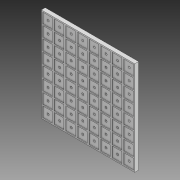
# Autodesk Inventor part: Solenoid Plate
Saved by Autodesk Inventor 2020 (Build 240168000, 168)
## iProperties
Created: 2020-08-11
Part Number: Solenoid Plate
Material: Generic
Document SubType Name: Modeling
Designer: DDeGo
Density: 1 g/cm^3
Appearance: Default
Author: DDeGo
Autodesk Inventor part; units mm, degrees
ref_plane "YZ Plane" through (0, 0, 0) normal (1, 0, 0) x (0, 1, 0)
ref_plane "XZ Plane" through (0, 0, 0) normal (0, 1, 0) x (-1, 0, 0)
ref_plane "XY Plane" through (0, 0, 0) normal (0, 0, 1) x (1, 0, 0)
sketch "Sketch1" plane through (0, 0, 0) normal (0, 0, 1) x (1, 0, 0)
  line L0 (0, 0) -> (145, 0)
  line L1 (145, 0) -> (145, 146)
  line L2 (145, 146) -> (0, 146)
  line L3 (0, 146) -> (0, 0)
  line L4 (2, 2) -> (17, 2) construction
  line L5 (17, 2) -> (17, 18) construction
  line L6 (17, 18) -> (2, 18) construction
  line L7 (2, 18) -> (2, 2) construction
  line L8 (2, 2) -> (17, 18) construction
  line L9 (17, 2) -> (2, 18) construction
  circle A0 centre (9.5, 10) radius 1.6
  line L10 (20, 2) -> (35, 2) construction
  line L11 (35, 2) -> (35, 18) construction
  line L12 (35, 18) -> (20, 18) construction
  line L13 (20, 18) -> (20, 2) construction
  line L14 (20, 2) -> (35, 18) construction
  line L15 (35, 2) -> (20, 18) construction
  circle A1 centre (27.5, 10) radius 1.6
  line L16 (38, 2) -> (53, 2) construction
  line L17 (53, 2) -> (53, 18) construction
  line L18 (53, 18) -> (38, 18) construction
  line L19 (38, 18) -> (38, 2) construction
  line L20 (38, 2) -> (53, 18) construction
  line L21 (53, 2) -> (38, 18) construction
  circle A2 centre (45.5, 10) radius 1.6
  line L22 (56, 2) -> (71, 2) construction
  line L23 (71, 2) -> (71, 18) construction
  line L24 (71, 18) -> (56, 18) construction
  line L25 (56, 18) -> (56, 2) construction
  line L26 (56, 2) -> (71, 18) construction
  line L27 (71, 2) -> (56, 18) construction
  circle A3 centre (63.5, 10) radius 1.6
  line L28 (74, 2) -> (89, 2) construction
  line L29 (89, 2) -> (89, 18) construction
  line L30 (89, 18) -> (74, 18) construction
  line L31 (74, 18) -> (74, 2) construction
  line L32 (74, 2) -> (89, 18) construction
  line L33 (89, 2) -> (74, 18) construction
  circle A4 centre (81.5, 10) radius 1.6
  line L34 (92, 2) -> (107, 2) construction
  line L35 (107, 2) -> (107, 18) construction
  line L36 (107, 18) -> (92, 18) construction
  line L37 (92, 18) -> (92, 2) construction
  line L38 (92, 2) -> (107, 18) construction
  line L39 (107, 2) -> (92, 18) construction
  circle A5 centre (99.5, 10) radius 1.6
  line L40 (110, 2) -> (125, 2) construction
  line L41 (125, 2) -> (125, 18) construction
  line L42 (125, 18) -> (110, 18) construction
  line L43 (110, 18) -> (110, 2) construction
  line L44 (110, 2) -> (125, 18) construction
  line L45 (125, 2) -> (110, 18) construction
  circle A6 centre (117.5, 10) radius 1.6
  line L46 (128, 2) -> (143, 2) construction
  line L47 (143, 2) -> (143, 18) construction
  line L48 (143, 18) -> (128, 18) construction
  line L49 (128, 18) -> (128, 2) construction
  line L50 (128, 2) -> (143, 18) construction
  line L51 (143, 2) -> (128, 18) construction
  circle A7 centre (135.5, 10) radius 1.6
  line L52 (2, 20) -> (17, 20) construction
  line L53 (17, 20) -> (17, 36) construction
  line L54 (17, 36) -> (2, 36) construction
  line L55 (2, 36) -> (2, 20) construction
  line L56 (2, 20) -> (17, 36) construction
  line L57 (17, 20) -> (2, 36) construction
  circle A8 centre (9.5, 28) radius 1.6
  line L58 (20, 20) -> (35, 20) construction
  line L59 (35, 20) -> (35, 36) construction
  line L60 (35, 36) -> (20, 36) construction
  line L61 (20, 36) -> (20, 20) construction
  line L62 (20, 20) -> (35, 36) construction
  line L63 (35, 20) -> (20, 36) construction
  circle A9 centre (27.5, 28) radius 1.6
  line L64 (38, 20) -> (53, 20) construction
  line L65 (53, 20) -> (53, 36) construction
  line L66 (53, 36) -> (38, 36) construction
  line L67 (38, 36) -> (38, 20) construction
  line L68 (38, 20) -> (53, 36) construction
  line L69 (53, 20) -> (38, 36) construction
  circle A10 centre (45.5, 28) radius 1.6
  line L70 (56, 20) -> (71, 20) construction
  line L71 (71, 20) -> (71, 36) construction
  line L72 (71, 36) -> (56, 36) construction
  line L73 (56, 36) -> (56, 20) construction
  line L74 (56, 20) -> (71, 36) construction
  line L75 (71, 20) -> (56, 36) construction
  circle A11 centre (63.5, 28) radius 1.6
  line L76 (74, 20) -> (89, 20) construction
  line L77 (89, 20) -> (89, 36) construction
  line L78 (89, 36) -> (74, 36) construction
  line L79 (74, 36) -> (74, 20) construction
  line L80 (74, 20) -> (89, 36) construction
  line L81 (89, 20) -> (74, 36) construction
  circle A12 centre (81.5, 28) radius 1.6
  line L82 (92, 20) -> (107, 20) construction
  line L83 (107, 20) -> (107, 36) construction
  line L84 (107, 36) -> (92, 36) construction
  line L85 (92, 36) -> (92, 20) construction
  line L86 (92, 20) -> (107, 36) construction
  line L87 (107, 20) -> (92, 36) construction
  circle A13 centre (99.5, 28) radius 1.6
  line L88 (110, 20) -> (125, 20) construction
  line L89 (125, 20) -> (125, 36) construction
  line L90 (125, 36) -> (110, 36) construction
  line L91 (110, 36) -> (110, 20) construction
  line L92 (110, 20) -> (125, 36) construction
  line L93 (125, 20) -> (110, 36) construction
  circle A14 centre (117.5, 28) radius 1.6
  line L94 (128, 20) -> (143, 20) construction
  line L95 (143, 20) -> (143, 36) construction
  line L96 (143, 36) -> (128, 36) construction
  line L97 (128, 36) -> (128, 20) construction
  line L98 (128, 20) -> (143, 36) construction
  line L99 (143, 20) -> (128, 36) construction
  circle A15 centre (135.5, 28) radius 1.6
  line L100 (2, 38) -> (17, 38) construction
  line L101 (17, 38) -> (17, 54) construction
  line L102 (17, 54) -> (2, 54) construction
  line L103 (2, 54) -> (2, 38) construction
  line L104 (2, 38) -> (17, 54) construction
  line L105 (17, 38) -> (2, 54) construction
  circle A16 centre (9.5, 46) radius 1.6
  line L106 (20, 38) -> (35, 38) construction
  line L107 (35, 38) -> (35, 54) construction
  line L108 (35, 54) -> (20, 54) construction
  line L109 (20, 54) -> (20, 38) construction
  line L110 (20, 38) -> (35, 54) construction
  line L111 (35, 38) -> (20, 54) construction
  circle A17 centre (27.5, 46) radius 1.6
  line L112 (38, 38) -> (53, 38) construction
  line L113 (53, 38) -> (53, 54) construction
  line L114 (53, 54) -> (38, 54) construction
  line L115 (38, 54) -> (38, 38) construction
  line L116 (38, 38) -> (53, 54) construction
  line L117 (53, 38) -> (38, 54) construction
  circle A18 centre (45.5, 46) radius 1.6
  line L118 (56, 38) -> (71, 38) construction
  line L119 (71, 38) -> (71, 54) construction
  line L120 (71, 54) -> (56, 54) construction
  line L121 (56, 54) -> (56, 38) construction
  line L122 (56, 38) -> (71, 54) construction
  line L123 (71, 38) -> (56, 54) construction
  circle A19 centre (63.5, 46) radius 1.6
  line L124 (74, 38) -> (89, 38) construction
  line L125 (89, 38) -> (89, 54) construction
  line L126 (89, 54) -> (74, 54) construction
  line L127 (74, 54) -> (74, 38) construction
  line L128 (74, 38) -> (89, 54) construction
  line L129 (89, 38) -> (74, 54) construction
  circle A20 centre (81.5, 46) radius 1.6
  line L130 (92, 38) -> (107, 38) construction
  line L131 (107, 38) -> (107, 54) construction
  line L132 (107, 54) -> (92, 54) construction
  line L133 (92, 54) -> (92, 38) construction
  line L134 (92, 38) -> (107, 54) construction
  line L135 (107, 38) -> (92, 54) construction
  circle A21 centre (99.5, 46) radius 1.6
  line L136 (110, 38) -> (125, 38) construction
  line L137 (125, 38) -> (125, 54) construction
  line L138 (125, 54) -> (110, 54) construction
  line L139 (110, 54) -> (110, 38) construction
  line L140 (110, 38) -> (125, 54) construction
  line L141 (125, 38) -> (110, 54) construction
  circle A22 centre (117.5, 46) radius 1.6
  line L142 (128, 38) -> (143, 38) construction
  line L143 (143, 38) -> (143, 54) construction
  line L144 (143, 54) -> (128, 54) construction
  line L145 (128, 54) -> (128, 38) construction
  line L146 (128, 38) -> (143, 54) construction
  line L147 (143, 38) -> (128, 54) construction
  circle A23 centre (135.5, 46) radius 1.6
  line L148 (2, 56) -> (17, 56) construction
  line L149 (17, 56) -> (17, 72) construction
  line L150 (17, 72) -> (2, 72) construction
  line L151 (2, 72) -> (2, 56) construction
  line L152 (2, 56) -> (17, 72) construction
  line L153 (17, 56) -> (2, 72) construction
  circle A24 centre (9.5, 64) radius 1.6
  line L154 (20, 56) -> (35, 56) construction
  line L155 (35, 56) -> (35, 72) construction
  line L156 (35, 72) -> (20, 72) construction
  line L157 (20, 72) -> (20, 56) construction
  line L158 (20, 56) -> (35, 72) construction
  line L159 (35, 56) -> (20, 72) construction
  circle A25 centre (27.5, 64) radius 1.6
  line L160 (38, 56) -> (53, 56) construction
  line L161 (53, 56) -> (53, 72) construction
  line L162 (53, 72) -> (38, 72) construction
  line L163 (38, 72) -> (38, 56) construction
  line L164 (38, 56) -> (53, 72) construction
  line L165 (53, 56) -> (38, 72) construction
  circle A26 centre (45.5, 64) radius 1.6
  line L166 (56, 56) -> (71, 56) construction
  line L167 (71, 56) -> (71, 72) construction
  line L168 (71, 72) -> (56, 72) construction
  line L169 (56, 72) -> (56, 56) construction
  line L170 (56, 56) -> (71, 72) construction
  line L171 (71, 56) -> (56, 72) construction
  circle A27 centre (63.5, 64) radius 1.6
  line L172 (74, 56) -> (89, 56) construction
  line L173 (89, 56) -> (89, 72) construction
  line L174 (89, 72) -> (74, 72) construction
  line L175 (74, 72) -> (74, 56) construction
  line L176 (74, 56) -> (89, 72) construction
  line L177 (89, 56) -> (74, 72) construction
  circle A28 centre (81.5, 64) radius 1.6
  line L178 (92, 56) -> (107, 56) construction
  line L179 (107, 56) -> (107, 72) construction
  line L180 (107, 72) -> (92, 72) construction
  line L181 (92, 72) -> (92, 56) construction
  line L182 (92, 56) -> (107, 72) construction
  line L183 (107, 56) -> (92, 72) construction
  circle A29 centre (99.5, 64) radius 1.6
  line L184 (110, 56) -> (125, 56) construction
  line L185 (125, 56) -> (125, 72) construction
  line L186 (125, 72) -> (110, 72) construction
  line L187 (110, 72) -> (110, 56) construction
  line L188 (110, 56) -> (125, 72) construction
  line L189 (125, 56) -> (110, 72) construction
  circle A30 centre (117.5, 64) radius 1.6
  line L190 (128, 56) -> (143, 56) construction
  line L191 (143, 56) -> (143, 72) construction
  line L192 (143, 72) -> (128, 72) construction
  line L193 (128, 72) -> (128, 56) construction
  line L194 (128, 56) -> (143, 72) construction
  line L195 (143, 56) -> (128, 72) construction
  circle A31 centre (135.5, 64) radius 1.6
  line L196 (2, 74) -> (17, 74) construction
  line L197 (17, 74) -> (17, 90) construction
  line L198 (17, 90) -> (2, 90) construction
  line L199 (2, 90) -> (2, 74) construction
  line L200 (2, 74) -> (17, 90) construction
  line L201 (17, 74) -> (2, 90) construction
  circle A32 centre (9.5, 82) radius 1.6
  line L202 (20, 74) -> (35, 74) construction
  line L203 (35, 74) -> (35, 90) construction
  line L204 (35, 90) -> (20, 90) construction
  line L205 (20, 90) -> (20, 74) construction
  line L206 (20, 74) -> (35, 90) construction
  line L207 (35, 74) -> (20, 90) construction
  circle A33 centre (27.5, 82) radius 1.6
  line L208 (38, 74) -> (53, 74) construction
  line L209 (53, 74) -> (53, 90) construction
  line L210 (53, 90) -> (38, 90) construction
  line L211 (38, 90) -> (38, 74) construction
  line L212 (38, 74) -> (53, 90) construction
  line L213 (53, 74) -> (38, 90) construction
  circle A34 centre (45.5, 82) radius 1.6
  line L214 (56, 74) -> (71, 74) construction
  line L215 (71, 74) -> (71, 90) construction
  line L216 (71, 90) -> (56, 90) construction
  line L217 (56, 90) -> (56, 74) construction
  line L218 (56, 74) -> (71, 90) construction
  line L219 (71, 74) -> (56, 90) construction
  circle A35 centre (63.5, 82) radius 1.6
  line L220 (74, 74) -> (89, 74) construction
  line L221 (89, 74) -> (89, 90) construction
  line L222 (89, 90) -> (74, 90) construction
  line L223 (74, 90) -> (74, 74) construction
  line L224 (74, 74) -> (89, 90) construction
  line L225 (89, 74) -> (74, 90) construction
  circle A36 centre (81.5, 82) radius 1.6
  line L226 (92, 74) -> (107, 74) construction
  line L227 (107, 74) -> (107, 90) construction
  line L228 (107, 90) -> (92, 90) construction
  line L229 (92, 90) -> (92, 74) construction
  line L230 (92, 74) -> (107, 90) construction
  line L231 (107, 74) -> (92, 90) construction
  circle A37 centre (99.5, 82) radius 1.6
  line L232 (110, 74) -> (125, 74) construction
  line L233 (125, 74) -> (125, 90) construction
  line L234 (125, 90) -> (110, 90) construction
  line L235 (110, 90) -> (110, 74) construction
  line L236 (110, 74) -> (125, 90) construction
  line L237 (125, 74) -> (110, 90) construction
  circle A38 centre (117.5, 82) radius 1.6
  line L238 (128, 74) -> (143, 74) construction
  line L239 (143, 74) -> (143, 90) construction
  line L240 (143, 90) -> (128, 90) construction
  line L241 (128, 90) -> (128, 74) construction
  line L242 (128, 74) -> (143, 90) construction
  line L243 (143, 74) -> (128, 90) construction
  circle A39 centre (135.5, 82) radius 1.6
  line L244 (2, 92) -> (17, 92) construction
  line L245 (17, 92) -> (17, 108) construction
  line L246 (17, 108) -> (2, 108) construction
  line L247 (2, 108) -> (2, 92) construction
  line L248 (2, 92) -> (17, 108) construction
  line L249 (17, 92) -> (2, 108) construction
  circle A40 centre (9.5, 100) radius 1.6
  line L250 (20, 92) -> (35, 92) construction
  line L251 (35, 92) -> (35, 108) construction
  line L252 (35, 108) -> (20, 108) construction
  line L253 (20, 108) -> (20, 92) construction
  line L254 (20, 92) -> (35, 108) construction
  line L255 (35, 92) -> (20, 108) construction
  circle A41 centre (27.5, 100) radius 1.6
  line L256 (38, 92) -> (53, 92) construction
  line L257 (53, 92) -> (53, 108) construction
  line L258 (53, 108) -> (38, 108) construction
  line L259 (38, 108) -> (38, 92) construction
  line L260 (38, 92) -> (53, 108) construction
  line L261 (53, 92) -> (38, 108) construction
  circle A42 centre (45.5, 100) radius 1.6
  line L262 (56, 92) -> (71, 92) construction
  line L263 (71, 92) -> (71, 108) construction
  line L264 (71, 108) -> (56, 108) construction
  line L265 (56, 108) -> (56, 92) construction
  line L266 (56, 92) -> (71, 108) construction
  line L267 (71, 92) -> (56, 108) construction
  circle A43 centre (63.5, 100) radius 1.6
  line L268 (74, 92) -> (89, 92) construction
  line L269 (89, 92) -> (89, 108) construction
  line L270 (89, 108) -> (74, 108) construction
  line L271 (74, 108) -> (74, 92) construction
  line L272 (74, 92) -> (89, 108) construction
  line L273 (89, 92) -> (74, 108) construction
  circle A44 centre (81.5, 100) radius 1.6
  line L274 (92, 92) -> (107, 92) construction
  line L275 (107, 92) -> (107, 108) construction
  line L276 (107, 108) -> (92, 108) construction
  line L277 (92, 108) -> (92, 92) construction
  line L278 (92, 92) -> (107, 108) construction
  line L279 (107, 92) -> (92, 108) construction
  circle A45 centre (99.5, 100) radius 1.6
  line L280 (110, 92) -> (125, 92) construction
  line L281 (125, 92) -> (125, 108) construction
  line L282 (125, 108) -> (110, 108) construction
  line L283 (110, 108) -> (110, 92) construction
  line L284 (110, 92) -> (125, 108) construction
  line L285 (125, 92) -> (110, 108) construction
  circle A46 centre (117.5, 100) radius 1.6
  line L286 (128, 92) -> (143, 92) construction
  line L287 (143, 92) -> (143, 108) construction
  line L288 (143, 108) -> (128, 108) construction
  line L289 (128, 108) -> (128, 92) construction
  line L290 (128, 92) -> (143, 108) construction
  line L291 (143, 92) -> (128, 108) construction
  circle A47 centre (135.5, 100) radius 1.6
  line L292 (2, 110) -> (17, 110) construction
  line L293 (17, 110) -> (17, 126) construction
  line L294 (17, 126) -> (2, 126) construction
  line L295 (2, 126) -> (2, 110) construction
  line L296 (2, 110) -> (17, 126) construction
  line L297 (17, 110) -> (2, 126) construction
  circle A48 centre (9.5, 118) radius 1.6
  line L298 (20, 110) -> (35, 110) construction
  line L299 (35, 110) -> (35, 126) construction
  line L300 (35, 126) -> (20, 126) construction
  line L301 (20, 126) -> (20, 110) construction
  line L302 (20, 110) -> (35, 126) construction
  line L303 (35, 110) -> (20, 126) construction
  circle A49 centre (27.5, 118) radius 1.6
  line L304 (38, 110) -> (53, 110) construction
  line L305 (53, 110) -> (53, 126) construction
  line L306 (53, 126) -> (38, 126) construction
  line L307 (38, 126) -> (38, 110) construction
  line L308 (38, 110) -> (53, 126) construction
  line L309 (53, 110) -> (38, 126) construction
  circle A50 centre (45.5, 118) radius 1.6
  line L310 (56, 110) -> (71, 110) construction
  line L311 (71, 110) -> (71, 126) construction
  line L312 (71, 126) -> (56, 126) construction
  line L313 (56, 126) -> (56, 110) construction
  line L314 (56, 110) -> (71, 126) construction
  line L315 (71, 110) -> (56, 126) construction
  circle A51 centre (63.5, 118) radius 1.6
  line L316 (74, 110) -> (89, 110) construction
  line L317 (89, 110) -> (89, 126) construction
  line L318 (89, 126) -> (74, 126) construction
  line L319 (74, 126) -> (74, 110) construction
  line L320 (74, 110) -> (89, 126) construction
  line L321 (89, 110) -> (74, 126) construction
  circle A52 centre (81.5, 118) radius 1.6
  line L322 (92, 110) -> (107, 110) construction
  line L323 (107, 110) -> (107, 126) construction
  line L324 (107, 126) -> (92, 126) construction
  line L325 (92, 126) -> (92, 110) construction
  line L326 (92, 110) -> (107, 126) construction
  line L327 (107, 110) -> (92, 126) construction
  circle A53 centre (99.5, 118) radius 1.6
  line L328 (110, 110) -> (125, 110) construction
  line L329 (125, 110) -> (125, 126) construction
  line L330 (125, 126) -> (110, 126) construction
  line L331 (110, 126) -> (110, 110) construction
  line L332 (110, 110) -> (125, 126) construction
  line L333 (125, 110) -> (110, 126) construction
  circle A54 centre (117.5, 118) radius 1.6
  line L334 (128, 110) -> (143, 110) construction
  line L335 (143, 110) -> (143, 126) construction
  line L336 (143, 126) -> (128, 126) construction
  line L337 (128, 126) -> (128, 110) construction
  line L338 (128, 110) -> (143, 126) construction
  line L339 (143, 110) -> (128, 126) construction
  circle A55 centre (135.5, 118) radius 1.6
  line L340 (2, 128) -> (17, 128) construction
  line L341 (17, 128) -> (17, 144) construction
  line L342 (17, 144) -> (2, 144) construction
  line L343 (2, 144) -> (2, 128) construction
  line L344 (2, 128) -> (17, 144) construction
  line L345 (17, 128) -> (2, 144) construction
  circle A56 centre (9.5, 136) radius 1.6
  line L346 (20, 128) -> (35, 128) construction
  line L347 (35, 128) -> (35, 144) construction
  line L348 (35, 144) -> (20, 144) construction
  line L349 (20, 144) -> (20, 128) construction
  line L350 (20, 128) -> (35, 144) construction
  line L351 (35, 128) -> (20, 144) construction
  circle A57 centre (27.5, 136) radius 1.6
  line L352 (38, 128) -> (53, 128) construction
  line L353 (53, 128) -> (53, 144) construction
  line L354 (53, 144) -> (38, 144) construction
  line L355 (38, 144) -> (38, 128) construction
  line L356 (38, 128) -> (53, 144) construction
  line L357 (53, 128) -> (38, 144) construction
  circle A58 centre (45.5, 136) radius 1.6
  line L358 (56, 128) -> (71, 128) construction
  line L359 (71, 128) -> (71, 144) construction
  line L360 (71, 144) -> (56, 144) construction
  line L361 (56, 144) -> (56, 128) construction
  line L362 (56, 128) -> (71, 144) construction
  line L363 (71, 128) -> (56, 144) construction
  circle A59 centre (63.5, 136) radius 1.6
  line L364 (74, 128) -> (89, 128) construction
  line L365 (89, 128) -> (89, 144) construction
  line L366 (89, 144) -> (74, 144) construction
  line L367 (74, 144) -> (74, 128) construction
  line L368 (74, 128) -> (89, 144) construction
  line L369 (89, 128) -> (74, 144) construction
  circle A60 centre (81.5, 136) radius 1.6
  line L370 (92, 128) -> (107, 128) construction
  line L371 (107, 128) -> (107, 144) construction
  line L372 (107, 144) -> (92, 144) construction
  line L373 (92, 144) -> (92, 128) construction
  line L374 (92, 128) -> (107, 144) construction
  line L375 (107, 128) -> (92, 144) construction
  circle A61 centre (99.5, 136) radius 1.6
  line L376 (110, 128) -> (125, 128) construction
  line L377 (125, 128) -> (125, 144) construction
  line L378 (125, 144) -> (110, 144) construction
  line L379 (110, 144) -> (110, 128) construction
  line L380 (110, 128) -> (125, 144) construction
  line L381 (125, 128) -> (110, 144) construction
  circle A62 centre (117.5, 136) radius 1.6
  line L382 (128, 128) -> (143, 128) construction
  line L383 (143, 128) -> (143, 144) construction
  line L384 (143, 144) -> (128, 144) construction
  line L385 (128, 144) -> (128, 128) construction
  line L386 (128, 128) -> (143, 144) construction
  line L387 (143, 128) -> (128, 144) construction
  circle A63 centre (135.5, 136) radius 1.6
  point P0 (9.5, 10)
  point P1 (27.5, 10)
  point P2 (45.5, 10)
  point P3 (63.5, 10)
  point P4 (81.5, 10)
  point P5 (99.5, 10)
  point P6 (117.5, 10)
  point P7 (135.5, 10)
  point P8 (9.5, 28)
  point P9 (63.5, 28)
  point P10 (9.5, 46)
  point P11 (63.5, 46)
  point P12 (9.5, 64)
  point P13 (63.5, 64)
  point P14 (9.5, 82)
  point P15 (63.5, 82)
  point P16 (9.5, 100)
  point P17 (63.5, 100)
  point P18 (9.5, 118)
  point P19 (63.5, 118)
  point P20 (9.5, 136)
  point P21 (63.5, 136)
  dimension "d0" = 2
  dimension "d1" = 2
  dimension "d2" = 16
  dimension "d3" = 15
  dimension "d4" = 3.2
  dimension "d7" = 18
  dimension "d10" = 18
  dimension "d13" = 2
  dimension "d14" = 2
  dimension "d27" = 145
  dimension "d28" = 146
  constraints: 776 end point, 128 midpoint, 64 centre point, 64 coincident, 4 parallel, 3 horizontal, 2 perpendicular, 1 vertical, 819 other
  measures "d0" distance between parallel lines of L0 L4
  measures "d1" distance between parallel lines of L3 L7
  measures "d2" distance of L6.end L4.start
  measures "d3" distance of L4.start L4.end
  measures "d4" diameter of A0
  measures "d7" distance of L4.start L10.start
  measures "d10" distance of L4.start L52.start
  measures "d13" distance between parallel lines of L1 L47
  measures "d14" distance between parallel lines of L2 L342
  measures "d27" distance of L1.end L2.end
  measures "d28" distance of L0.end L1.end
extrude "Extrusion1" add sketch "Sketch1" along normal blind 6
sketch "Sketch2" plane through (0, 0, 6) normal (0, 0, 1) x (1, 0, 0)
  line L0 (2, 2) -> (17, 2)
  line L1 (17, 2) -> (17, 18)
  line L2 (17, 18) -> (2, 18)
  line L3 (2, 18) -> (2, 2)
  line L4 (2, 2) -> (17, 18) construction
  line L5 (17, 2) -> (2, 18) construction
  line L6 (20, 2) -> (35, 2)
  line L7 (35, 2) -> (35, 18)
  line L8 (35, 18) -> (20, 18)
  line L9 (20, 18) -> (20, 2)
  line L10 (20, 2) -> (35, 18) construction
  line L11 (35, 2) -> (20, 18) construction
  line L12 (2, 20) -> (17, 20)
  line L13 (17, 20) -> (17, 36)
  line L14 (17, 36) -> (2, 36)
  line L15 (2, 36) -> (2, 20)
  line L16 (2, 20) -> (17, 36) construction
  line L17 (17, 20) -> (2, 36) construction
  line L18 (20, 20) -> (35, 20)
  line L19 (35, 20) -> (35, 36)
  line L20 (35, 36) -> (20, 36)
  line L21 (20, 36) -> (20, 20)
  line L22 (20, 20) -> (35, 36) construction
  line L23 (35, 20) -> (20, 36) construction
  line L24 (38, 2) -> (53, 2)
  line L25 (53, 2) -> (53, 18)
  line L26 (53, 18) -> (38, 18)
  line L27 (38, 18) -> (38, 2)
  line L28 (38, 2) -> (53, 18) construction
  line L29 (53, 2) -> (38, 18) construction
  line L30 (38, 20) -> (53, 20)
  line L31 (53, 20) -> (53, 36)
  line L32 (53, 36) -> (38, 36)
  line L33 (38, 36) -> (38, 20)
  line L34 (38, 20) -> (53, 36) construction
  line L35 (53, 20) -> (38, 36) construction
  line L36 (56, 2) -> (71, 2)
  line L37 (71, 2) -> (71, 18)
  line L38 (71, 18) -> (56, 18)
  line L39 (56, 18) -> (56, 2)
  line L40 (56, 2) -> (71, 18) construction
  line L41 (71, 2) -> (56, 18) construction
  line L42 (56, 20) -> (71, 20)
  line L43 (71, 20) -> (71, 36)
  line L44 (71, 36) -> (56, 36)
  line L45 (56, 36) -> (56, 20)
  line L46 (56, 20) -> (71, 36) construction
  line L47 (71, 20) -> (56, 36) construction
  line L48 (74, 2) -> (89, 2)
  line L49 (89, 2) -> (89, 18)
  line L50 (89, 18) -> (74, 18)
  line L51 (74, 18) -> (74, 2)
  line L52 (74, 2) -> (89, 18) construction
  line L53 (89, 2) -> (74, 18) construction
  line L54 (74, 20) -> (89, 20)
  line L55 (89, 20) -> (89, 36)
  line L56 (89, 36) -> (74, 36)
  line L57 (74, 36) -> (74, 20)
  line L58 (74, 20) -> (89, 36) construction
  line L59 (89, 20) -> (74, 36) construction
  line L60 (92, 2) -> (107, 2)
  line L61 (107, 2) -> (107, 18)
  line L62 (107, 18) -> (92, 18)
  line L63 (92, 18) -> (92, 2)
  line L64 (92, 2) -> (107, 18) construction
  line L65 (107, 2) -> (92, 18) construction
  line L66 (92, 20) -> (107, 20)
  line L67 (107, 20) -> (107, 36)
  line L68 (107, 36) -> (92, 36)
  line L69 (92, 36) -> (92, 20)
  line L70 (92, 20) -> (107, 36) construction
  line L71 (107, 20) -> (92, 36) construction
  line L72 (110, 2) -> (125, 2)
  line L73 (125, 2) -> (125, 18)
  line L74 (125, 18) -> (110, 18)
  line L75 (110, 18) -> (110, 2)
  line L76 (110, 2) -> (125, 18) construction
  line L77 (125, 2) -> (110, 18) construction
  line L78 (110, 20) -> (125, 20)
  line L79 (125, 20) -> (125, 36)
  line L80 (125, 36) -> (110, 36)
  line L81 (110, 36) -> (110, 20)
  line L82 (110, 20) -> (125, 36) construction
  line L83 (125, 20) -> (110, 36) construction
  line L84 (128, 2) -> (143, 2)
  line L85 (143, 2) -> (143, 18)
  line L86 (143, 18) -> (128, 18)
  line L87 (128, 18) -> (128, 2)
  line L88 (128, 2) -> (143, 18) construction
  line L89 (143, 2) -> (128, 18) construction
  line L90 (128, 20) -> (143, 20)
  line L91 (143, 20) -> (143, 36)
  line L92 (143, 36) -> (128, 36)
  line L93 (128, 36) -> (128, 20)
  line L94 (128, 20) -> (143, 36) construction
  line L95 (143, 20) -> (128, 36) construction
  line L96 (2, 38) -> (17, 38)
  line L97 (17, 38) -> (17, 54)
  line L98 (17, 54) -> (2, 54)
  line L99 (2, 54) -> (2, 38)
  line L100 (2, 38) -> (17, 54) construction
  line L101 (17, 38) -> (2, 54) construction
  line L102 (20, 38) -> (35, 38)
  line L103 (35, 38) -> (35, 54)
  line L104 (35, 54) -> (20, 54)
  line L105 (20, 54) -> (20, 38)
  line L106 (20, 38) -> (35, 54) construction
  line L107 (35, 38) -> (20, 54) construction
  line L108 (38, 38) -> (53, 38)
  line L109 (53, 38) -> (53, 54)
  line L110 (53, 54) -> (38, 54)
  line L111 (38, 54) -> (38, 38)
  line L112 (38, 38) -> (53, 54) construction
  line L113 (53, 38) -> (38, 54) construction
  line L114 (56, 38) -> (71, 38)
  line L115 (71, 38) -> (71, 54)
  line L116 (71, 54) -> (56, 54)
  line L117 (56, 54) -> (56, 38)
  line L118 (56, 38) -> (71, 54) construction
  line L119 (71, 38) -> (56, 54) construction
  line L120 (74, 38) -> (89, 38)
  line L121 (89, 38) -> (89, 54)
  line L122 (89, 54) -> (74, 54)
  line L123 (74, 54) -> (74, 38)
  line L124 (74, 38) -> (89, 54) construction
  line L125 (89, 38) -> (74, 54) construction
  line L126 (92, 38) -> (107, 38)
  line L127 (107, 38) -> (107, 54)
  line L128 (107, 54) -> (92, 54)
  line L129 (92, 54) -> (92, 38)
  line L130 (92, 38) -> (107, 54) construction
  line L131 (107, 38) -> (92, 54) construction
  line L132 (110, 38) -> (125, 38)
  line L133 (125, 38) -> (125, 54)
  line L134 (125, 54) -> (110, 54)
  line L135 (110, 54) -> (110, 38)
  line L136 (110, 38) -> (125, 54) construction
  line L137 (125, 38) -> (110, 54) construction
  line L138 (128, 38) -> (143, 38)
  line L139 (143, 38) -> (143, 54)
  line L140 (143, 54) -> (128, 54)
  line L141 (128, 54) -> (128, 38)
  line L142 (128, 38) -> (143, 54) construction
  line L143 (143, 38) -> (128, 54) construction
  line L144 (2, 56) -> (17, 56)
  line L145 (17, 56) -> (17, 72)
  line L146 (17, 72) -> (2, 72)
  line L147 (2, 72) -> (2, 56)
  line L148 (2, 56) -> (17, 72) construction
  line L149 (17, 56) -> (2, 72) construction
  line L150 (20, 56) -> (35, 56)
  line L151 (35, 56) -> (35, 72)
  line L152 (35, 72) -> (20, 72)
  line L153 (20, 72) -> (20, 56)
  line L154 (20, 56) -> (35, 72) construction
  line L155 (35, 56) -> (20, 72) construction
  line L156 (38, 56) -> (53, 56)
  line L157 (53, 56) -> (53, 72)
  line L158 (53, 72) -> (38, 72)
  line L159 (38, 72) -> (38, 56)
  line L160 (38, 56) -> (53, 72) construction
  line L161 (53, 56) -> (38, 72) construction
  line L162 (56, 56) -> (71, 56)
  line L163 (71, 56) -> (71, 72)
  line L164 (71, 72) -> (56, 72)
  line L165 (56, 72) -> (56, 56)
  line L166 (56, 56) -> (71, 72) construction
  line L167 (71, 56) -> (56, 72) construction
  line L168 (74, 56) -> (89, 56)
  line L169 (89, 56) -> (89, 72)
  line L170 (89, 72) -> (74, 72)
  line L171 (74, 72) -> (74, 56)
  line L172 (74, 56) -> (89, 72) construction
  line L173 (89, 56) -> (74, 72) construction
  line L174 (92, 56) -> (107, 56)
  line L175 (107, 56) -> (107, 72)
  line L176 (107, 72) -> (92, 72)
  line L177 (92, 72) -> (92, 56)
  line L178 (92, 56) -> (107, 72) construction
  line L179 (107, 56) -> (92, 72) construction
  line L180 (110, 56) -> (125, 56)
  line L181 (125, 56) -> (125, 72)
  line L182 (125, 72) -> (110, 72)
  line L183 (110, 72) -> (110, 56)
  line L184 (110, 56) -> (125, 72) construction
  line L185 (125, 56) -> (110, 72) construction
  line L186 (128, 56) -> (143, 56)
  line L187 (143, 56) -> (143, 72)
  line L188 (143, 72) -> (128, 72)
  line L189 (128, 72) -> (128, 56)
  line L190 (128, 56) -> (143, 72) construction
  line L191 (143, 56) -> (128, 72) construction
  line L192 (2, 74) -> (17, 74)
  line L193 (17, 74) -> (17, 90)
  line L194 (17, 90) -> (2, 90)
  line L195 (2, 90) -> (2, 74)
  line L196 (2, 74) -> (17, 90) construction
  line L197 (17, 74) -> (2, 90) construction
  line L198 (20, 74) -> (35, 74)
  line L199 (35, 74) -> (35, 90)
  line L200 (35, 90) -> (20, 90)
  line L201 (20, 90) -> (20, 74)
  line L202 (20, 74) -> (35, 90) construction
  line L203 (35, 74) -> (20, 90) construction
  line L204 (38, 74) -> (53, 74)
  line L205 (53, 74) -> (53, 90)
  line L206 (53, 90) -> (38, 90)
  line L207 (38, 90) -> (38, 74)
  line L208 (38, 74) -> (53, 90) construction
  line L209 (53, 74) -> (38, 90) construction
  line L210 (56, 74) -> (71, 74)
  line L211 (71, 74) -> (71, 90)
  line L212 (71, 90) -> (56, 90)
  line L213 (56, 90) -> (56, 74)
  line L214 (56, 74) -> (71, 90) construction
  line L215 (71, 74) -> (56, 90) construction
  line L216 (74, 74) -> (89, 74)
  line L217 (89, 74) -> (89, 90)
  line L218 (89, 90) -> (74, 90)
  line L219 (74, 90) -> (74, 74)
  line L220 (74, 74) -> (89, 90) construction
  line L221 (89, 74) -> (74, 90) construction
  line L222 (92, 74) -> (107, 74)
  line L223 (107, 74) -> (107, 90)
  line L224 (107, 90) -> (92, 90)
  line L225 (92, 90) -> (92, 74)
  line L226 (92, 74) -> (107, 90) construction
  line L227 (107, 74) -> (92, 90) construction
  line L228 (110, 74) -> (125, 74)
  line L229 (125, 74) -> (125, 90)
  line L230 (125, 90) -> (110, 90)
  line L231 (110, 90) -> (110, 74)
  line L232 (110, 74) -> (125, 90) construction
  line L233 (125, 74) -> (110, 90) construction
  line L234 (128, 74) -> (143, 74)
  line L235 (143, 74) -> (143, 90)
  line L236 (143, 90) -> (128, 90)
  line L237 (128, 90) -> (128, 74)
  line L238 (128, 74) -> (143, 90) construction
  line L239 (143, 74) -> (128, 90) construction
  line L240 (2, 92) -> (17, 92)
  line L241 (17, 92) -> (17, 108)
  line L242 (17, 108) -> (2, 108)
  line L243 (2, 108) -> (2, 92)
  line L244 (2, 92) -> (17, 108) construction
  line L245 (17, 92) -> (2, 108) construction
  line L246 (20, 92) -> (35, 92)
  line L247 (35, 92) -> (35, 108)
  line L248 (35, 108) -> (20, 108)
  line L249 (20, 108) -> (20, 92)
  line L250 (20, 92) -> (35, 108) construction
  line L251 (35, 92) -> (20, 108) construction
  line L252 (38, 92) -> (53, 92)
  line L253 (53, 92) -> (53, 108)
  line L254 (53, 108) -> (38, 108)
  line L255 (38, 108) -> (38, 92)
  line L256 (38, 92) -> (53, 108) construction
  line L257 (53, 92) -> (38, 108) construction
  line L258 (56, 92) -> (71, 92)
  line L259 (71, 92) -> (71, 108)
  line L260 (71, 108) -> (56, 108)
  line L261 (56, 108) -> (56, 92)
  line L262 (56, 92) -> (71, 108) construction
  line L263 (71, 92) -> (56, 108) construction
  line L264 (74, 92) -> (89, 92)
  line L265 (89, 92) -> (89, 108)
  line L266 (89, 108) -> (74, 108)
  line L267 (74, 108) -> (74, 92)
  line L268 (74, 92) -> (89, 108) construction
  line L269 (89, 92) -> (74, 108) construction
  line L270 (92, 92) -> (107, 92)
  line L271 (107, 92) -> (107, 108)
  line L272 (107, 108) -> (92, 108)
  line L273 (92, 108) -> (92, 92)
  line L274 (92, 92) -> (107, 108) construction
  line L275 (107, 92) -> (92, 108) construction
  line L276 (110, 92) -> (125, 92)
  line L277 (125, 92) -> (125, 108)
  line L278 (125, 108) -> (110, 108)
  line L279 (110, 108) -> (110, 92)
  line L280 (110, 92) -> (125, 108) construction
  line L281 (125, 92) -> (110, 108) construction
  line L282 (128, 92) -> (143, 92)
  line L283 (143, 92) -> (143, 108)
  line L284 (143, 108) -> (128, 108)
  line L285 (128, 108) -> (128, 92)
  line L286 (128, 92) -> (143, 108) construction
  line L287 (143, 92) -> (128, 108) construction
  line L288 (2, 110) -> (17, 110)
  line L289 (17, 110) -> (17, 126)
  line L290 (17, 126) -> (2, 126)
  line L291 (2, 126) -> (2, 110)
  line L292 (2, 110) -> (17, 126) construction
  line L293 (17, 110) -> (2, 126) construction
  line L294 (20, 110) -> (35, 110)
  line L295 (35, 110) -> (35, 126)
  line L296 (35, 126) -> (20, 126)
  line L297 (20, 126) -> (20, 110)
  line L298 (20, 110) -> (35, 126) construction
  line L299 (35, 110) -> (20, 126) construction
  line L300 (38, 110) -> (53, 110)
  line L301 (53, 110) -> (53, 126)
  line L302 (53, 126) -> (38, 126)
  line L303 (38, 126) -> (38, 110)
  line L304 (38, 110) -> (53, 126) construction
  line L305 (53, 110) -> (38, 126) construction
  line L306 (56, 110) -> (71, 110)
  line L307 (71, 110) -> (71, 126)
  line L308 (71, 126) -> (56, 126)
  line L309 (56, 126) -> (56, 110)
  line L310 (56, 110) -> (71, 126) construction
  line L311 (71, 110) -> (56, 126) construction
  line L312 (74, 110) -> (89, 110)
  line L313 (89, 110) -> (89, 126)
  line L314 (89, 126) -> (74, 126)
  line L315 (74, 126) -> (74, 110)
  line L316 (74, 110) -> (89, 126) construction
  line L317 (89, 110) -> (74, 126) construction
  line L318 (92, 110) -> (107, 110)
  line L319 (107, 110) -> (107, 126)
  line L320 (107, 126) -> (92, 126)
  line L321 (92, 126) -> (92, 110)
  line L322 (92, 110) -> (107, 126) construction
  line L323 (107, 110) -> (92, 126) construction
  line L324 (110, 110) -> (125, 110)
  line L325 (125, 110) -> (125, 126)
  line L326 (125, 126) -> (110, 126)
  line L327 (110, 126) -> (110, 110)
  line L328 (110, 110) -> (125, 126) construction
  line L329 (125, 110) -> (110, 126) construction
  line L330 (128, 110) -> (143, 110)
  line L331 (143, 110) -> (143, 126)
  line L332 (143, 126) -> (128, 126)
  line L333 (128, 126) -> (128, 110)
  line L334 (128, 110) -> (143, 126) construction
  line L335 (143, 110) -> (128, 126) construction
  line L336 (2, 128) -> (17, 128)
  line L337 (17, 128) -> (17, 144)
  line L338 (17, 144) -> (2, 144)
  line L339 (2, 144) -> (2, 128)
  line L340 (2, 128) -> (17, 144) construction
  line L341 (17, 128) -> (2, 144) construction
  line L342 (20, 128) -> (35, 128)
  line L343 (35, 128) -> (35, 144)
  line L344 (35, 144) -> (20, 144)
  line L345 (20, 144) -> (20, 128)
  line L346 (20, 128) -> (35, 144) construction
  line L347 (35, 128) -> (20, 144) construction
  line L348 (38, 128) -> (53, 128)
  line L349 (53, 128) -> (53, 144)
  line L350 (53, 144) -> (38, 144)
  line L351 (38, 144) -> (38, 128)
  line L352 (38, 128) -> (53, 144) construction
  line L353 (53, 128) -> (38, 144) construction
  line L354 (56, 128) -> (71, 128)
  line L355 (71, 128) -> (71, 144)
  line L356 (71, 144) -> (56, 144)
  line L357 (56, 144) -> (56, 128)
  line L358 (56, 128) -> (71, 144) construction
  line L359 (71, 128) -> (56, 144) construction
  line L360 (74, 128) -> (89, 128)
  line L361 (89, 128) -> (89, 144)
  line L362 (89, 144) -> (74, 144)
  line L363 (74, 144) -> (74, 128)
  line L364 (74, 128) -> (89, 144) construction
  line L365 (89, 128) -> (74, 144) construction
  line L366 (92, 128) -> (107, 128)
  line L367 (107, 128) -> (107, 144)
  line L368 (107, 144) -> (92, 144)
  line L369 (92, 144) -> (92, 128)
  line L370 (92, 128) -> (107, 144) construction
  line L371 (107, 128) -> (92, 144) construction
  line L372 (110, 128) -> (125, 128)
  line L373 (125, 128) -> (125, 144)
  line L374 (125, 144) -> (110, 144)
  line L375 (110, 144) -> (110, 128)
  line L376 (110, 128) -> (125, 144) construction
  line L377 (125, 128) -> (110, 144) construction
  line L378 (128, 128) -> (143, 128)
  line L379 (143, 128) -> (143, 144)
  line L380 (143, 144) -> (128, 144)
  line L381 (128, 144) -> (128, 128)
  line L382 (128, 128) -> (143, 144) construction
  line L383 (143, 128) -> (128, 144) construction
  point P0 (9.5, 10)
  point P1 (2, 18)
  point P2 (17, 2)
  point P3 (2, 2)
  point P4 (27.5, 10)
  point P5 (20, 18)
  point P6 (35, 2)
  point P7 (20, 2)
  point P8 (9.5, 28)
  point P9 (2, 36)
  point P10 (17, 20)
  point P11 (2, 20)
  point P12 (27.5, 28)
  point P13 (35, 20)
  point P14 (20, 20)
  point P15 (45.5, 10)
  point P16 (38, 18)
  point P17 (53, 2)
  point P18 (38, 2)
  point P19 (45.5, 28)
  point P20 (38, 36)
  point P21 (53, 20)
  point P22 (38, 20)
  point P23 (63.5, 10)
  point P24 (56, 18)
  point P25 (71, 2)
  point P26 (56, 2)
  point P27 (63.5, 28)
  point P28 (71, 20)
  point P29 (56, 20)
  point P30 (81.5, 10)
  point P31 (74, 18)
  point P32 (89, 2)
  point P33 (74, 2)
  point P34 (81.5, 28)
  point P35 (89, 20)
  point P36 (74, 20)
  point P37 (99.5, 10)
  point P38 (92, 18)
  point P39 (107, 2)
  point P40 (92, 2)
  point P41 (99.5, 28)
  point P42 (107, 20)
  point P43 (92, 20)
  point P44 (117.5, 10)
  point P45 (110, 18)
  point P46 (125, 2)
  point P47 (110, 2)
  point P48 (117.5, 28)
  point P49 (125, 20)
  point P50 (110, 20)
  point P51 (135.5, 10)
  point P52 (128, 18)
  point P53 (143, 2)
  point P54 (128, 2)
  point P55 (135.5, 28)
  point P56 (143, 20)
  point P57 (128, 20)
  point P58 (9.5, 46)
  point P59 (2, 54)
  point P60 (17, 38)
  point P61 (2, 38)
  point P62 (27.5, 46)
  point P63 (20, 54)
  point P64 (35, 38)
  point P65 (20, 38)
  point P66 (45.5, 46)
  point P67 (38, 54)
  point P68 (53, 38)
  point P69 (38, 38)
  point P70 (63.5, 46)
  point P71 (56, 54)
  point P72 (71, 38)
  point P73 (56, 38)
  point P74 (81.5, 46)
  point P75 (74, 54)
  point P76 (89, 38)
  point P77 (74, 38)
  point P78 (99.5, 46)
  point P79 (92, 54)
  point P80 (107, 38)
  point P81 (92, 38)
  point P82 (117.5, 46)
  point P83 (110, 54)
  point P84 (125, 38)
  point P85 (110, 38)
  point P86 (135.5, 46)
  point P87 (128, 54)
  point P88 (143, 38)
  point P89 (128, 38)
  point P90 (9.5, 64)
  point P91 (2, 72)
  point P92 (17, 56)
  point P93 (2, 56)
  point P94 (27.5, 64)
  point P95 (35, 56)
  point P96 (20, 56)
  point P97 (45.5, 64)
  point P98 (38, 72)
  point P99 (53, 56)
  point P100 (38, 56)
  point P101 (63.5, 64)
  point P102 (71, 56)
  point P103 (56, 56)
  point P104 (81.5, 64)
  point P105 (89, 56)
  point P106 (74, 56)
  point P107 (99.5, 64)
  point P108 (107, 56)
  point P109 (92, 56)
  point P110 (117.5, 64)
  point P111 (125, 56)
  point P112 (110, 56)
  point P113 (135.5, 64)
  point P114 (143, 56)
  point P115 (128, 56)
  point P116 (9.5, 82)
  point P117 (2, 90)
  point P118 (17, 74)
  point P119 (2, 74)
  point P120 (27.5, 82)
  point P121 (35, 74)
  point P122 (20, 74)
  point P123 (45.5, 82)
  point P124 (38, 90)
  point P125 (53, 74)
  point P126 (38, 74)
  point P127 (63.5, 82)
  point P128 (71, 74)
  point P129 (56, 74)
  point P130 (81.5, 82)
  point P131 (89, 74)
  point P132 (74, 74)
  point P133 (99.5, 82)
  point P134 (107, 74)
  point P135 (92, 74)
  point P136 (117.5, 82)
  point P137 (125, 74)
  point P138 (110, 74)
  point P139 (135.5, 82)
  point P140 (143, 74)
  point P141 (128, 74)
  point P142 (9.5, 100)
  point P143 (2, 108)
  point P144 (17, 92)
  point P145 (2, 92)
  point P146 (27.5, 100)
  point P147 (20, 92)
  point P148 (45.5, 100)
  point P149 (38, 108)
  point P150 (63.5, 100)
  point P151 (56, 92)
  point P152 (81.5, 100)
  point P153 (99.5, 100)
  point P154 (117.5, 100)
  point P155 (135.5, 100)
  point P156 (9.5, 118)
  point P157 (2, 126)
  point P158 (17, 110)
  point P159 (2, 110)
  point P160 (27.5, 118)
  point P161 (20, 110)
  point P162 (45.5, 118)
  point P163 (38, 126)
  point P164 (63.5, 118)
  point P165 (56, 110)
  point P166 (81.5, 118)
  point P167 (99.5, 118)
  point P168 (117.5, 118)
  point P169 (135.5, 118)
  point P170 (9.5, 136)
  point P171 (2, 144)
  point P172 (17, 128)
  point P173 (2, 128)
  point P174 (27.5, 136)
  point P175 (20, 128)
  point P176 (45.5, 136)
  point P177 (38, 144)
  point P178 (63.5, 136)
  point P179 (56, 128)
  point P180 (81.5, 136)
  point P181 (99.5, 136)
  point P182 (117.5, 136)
  point P183 (135.5, 136)
  dimension "d19" = 18
  dimension "d22" = 18
  constraints: 768 end point, 128 midpoint, 2 collinear, 2 horizontal, 2 parallel, 1 perpendicular, 1 vertical, 880 other
  measures "d19" distance of L0.start L6.start
  measures "d22" distance of L0.start L12.start
extrude "Extrusion2" cut sketch "Sketch2" against normal blind 1
equation "\"d1\" = d0"
equation "\"d13\" = d0"
equation "\"d14\" = d0"
equation "\"d19\" = d7"
equation "\"d22\" = d10"
body "Solid1"
